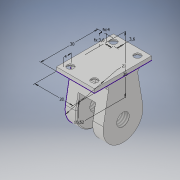
# Autodesk Inventor part: BT103_trajan20_21
Saved by Autodesk Inventor 2022.2 (Build 262287000, 287)
## iProperties
Company: HTBLA Kaindorf
RuleStatus: InUse
Created: 2022-08-02
Part Number: BT103_trajan20_21
Project: Zeichenmaschine_v2
Material: Generisch
Description: halterung2
Document SubType Name: Modeling
Designer: trajan20
Density: 1 g/cm^3
Appearance: Vorgabe
Mass: 8.17969 g
Surface Area: 40.6698 cm^2
Volume: 8.17969 cm^3
AfterDocNew0: iProperties-Editor_aufrufen
Author: jan
Keywords: 2021
Autodesk Inventor part; units mm, degrees
ref_plane "YZ Plane" through (0, 0, 0) normal (1, 0, 0) x (0, 1, 0)
ref_plane "XZ Plane" through (0, 0, 0) normal (0, 1, 0) x (-1, 0, 0)
ref_plane "XY Plane" through (0, 0, 0) normal (0, 0, 1) x (1, 0, 0)
sketch "Skizze3" plane through (0, 0, 0) normal (0, 0, 1) x (1, 0, 0)
  line L0 (0, 0) -> (30, 0)
  line L1 (30, 0) -> (30, 20)
  line L2 (30, 20) -> (0, 20)
  line L3 (0, 20) -> (0, 0)
  point P0 (3.6, 3.6)
  dimension "d4" = 30
  dimension "d5" = 20
  dimension "d6" = 3.6
  dimension "d7" = 3.6
  constraints: 8 end point, 2 parallel, 1 horizontal, 1 perpendicular
  measures "d4" distance between parallel lines of L3 L1
  measures "d5" distance between parallel lines of L2 L0
  measures "d6" distance from line of L3 point (3.6, 3.6)
  measures "d7" distance from line of L0 point (3.6, 3.6)
extrude "Extrusion3" add sketch "Skizze3" along normal blind 2
hole "Bohrung1" at (3.6, 3.6, 0) direction (0, 0, 1) diameter 3.5 depth 4 countersink diameter 6.5 countersink angle 90
pattern_linear "Rechteckige Anordnung1" count 2 spacing 12.6 along (0, 1, 0) count 2 spacing 22.6 along (1, 0, 0) of "Bohrung1"
sketch "Skizze4" plane through (0, 0, 0) normal (0, -1, 0) x (1, 0, 0)
  line L0 (29.45, 0) -> (22.95, 0) projected
  line L1 (6.85, 0) -> (0.35, 0) projected
  line L2 (0, 0) -> (30, 0) projected
  line L3 (22.2, 0) -> (25.3378, -17.6413)
  line L4 (7.6, 0) -> (4.6427, -17.7549)
  line L5 (30, 0) -> (0, 0) projected
  line L6 (15, 0) -> (15, -30)
  circle A0 centre (15, -19.48) radius 10.5
  point P0 (26.2, 0)
  point P1 (3.6, 0)
  dimension "d23" = 4
  dimension "d24" = 4
  dimension "d28" = 21
  dimension "d29" = 30
  dimension "d30" = 10.52
  constraints: 6 end point, 3 point on line, 2 midpoint, 2 point on circle, 2 tangent, 1 centre point, 1 perpendicular, 2 other
  measures "d23" distance of point (26.2, 0) L3.start
  measures "d24" distance of point (3.6, 0) L4.start
  measures "d28" diameter of A0
  measures "d29" distance of L6.start L6.end
  measures "d30" distance of L6.end A0.centre
extrude "Extrusion4" add sketch "Skizze4" against normal blind 20
hole "Bohrung2" at (15, 0, -19.48) direction (0, 1, 0) diameter 6.647 end through all thread size "M8x1.25" class "6H" standard "ISO Metric profile"
fillet "Rundung1" radius 2 2 edges at (7.6, 10, 0) (22.2, 10, 0)
sketch "Skizze5" plane through (30, 0, 0) normal (1, 0, 0) x (0, 0, -1)
  line L0 (29.98, 0) -> (29.98, 20) projected
  line L1 (29.98, 14.1) -> (9.98, 14.1)
  line L2 (9.98, 14.1) -> (9.98, 5.9)
  line L3 (9.98, 5.9) -> (29.98, 5.9)
  line L4 (29.98, 5.9) -> (29.98, 14.1)
  point P0 (0, 0)
  point P1 (29.98, 10)
  dimension "d42" = 8.2
  dimension "d43" = 20
  constraints: 8 end point, 2 midpoint, 2 parallel, 1 horizontal, 1 perpendicular, 1 point on line
  measures "d42" distance between parallel lines of L3 L1
  measures "d43" distance between parallel lines of L0 L2
extrude "Extrusion5" cut sketch "Skizze5" against normal through all
chamfer "Fase1" distance 0.5 angle 45 6 edges at (15.0576, 14.1, -29.9798) (5.2902, 14.1, -13.8674) (24.6564, 14.1, -13.8106) (15.0576, 5.9, -29.9798) (24.6564, 5.9, -13.8106) (5.2902, 5.9, -13.8674)
equation "\"d7\" = d6"
equation "\"d24\" = d23"
